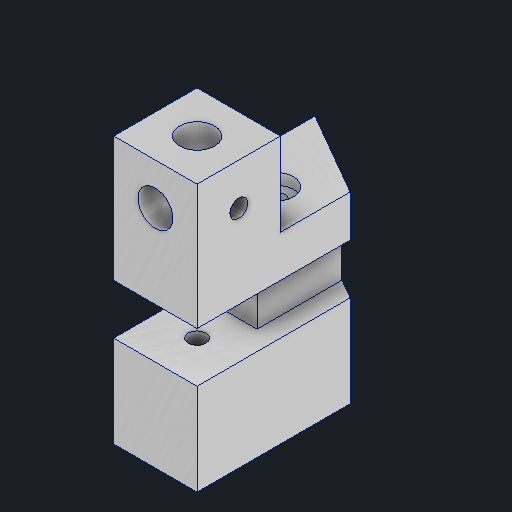
# Autodesk Inventor part: B Idler
Saved by Autodesk Inventor 2025.1 (Build 291241020, 241B)
## iProperties
Created: 2025-04-15
Part Number: B Idler
Material: Aluminum 6061
Document SubType Name: Modeling
Designer: Joshua Eah
Density: 2.7 g/cm^3
Appearance: Aluminum - Flat
Author: Joshua Eah
Autodesk Inventor part; units mm, degrees
ref_plane "YZ Plane" through (0, 0, 0) normal (1, 0, 0) x (0, 1, 0)
ref_plane "XZ Plane" through (0, 0, 0) normal (0, 1, 0) x (-1, 0, 0)
ref_plane "XY Plane" through (0, 0, 0) normal (0, 0, 1) x (1, 0, 0)
sketch "Sketch1" plane through (0, 0, 0) normal (0, 1, 0) x (-1, 0, 0)
  line L0 (0, 0) -> (-15, 0)
  line L1 (-15, 0) -> (-15, -36.2103)
  line L2 (-15, -36.2103) -> (0, -36.2103)
  line L3 (0, -36.2103) -> (0, 0)
  dimension "d0" = 15
  dimension "d1" = 36.2103
  constraints: 8 end point, 2 parallel, 1 horizontal, 1 perpendicular
  measures "d0" distance of L2.end L1.end
  measures "d1" distance of L1.end L0.end
extrude "Extrusion1" add sketch "Sketch1" along normal blind 48
sketch "Sketch2" plane through (0, 0, 0) normal (0, 0, 1) x (1, 0, 0)
  line L0 (0, 0) -> (15, 0) projected
  line L1 (15, 0) -> (15, 48) projected
  line L2 (0, 48) -> (15, 48) projected
  line L3 (0, 0) -> (0, 48) projected
  line L4 (0, 16.5) -> (3.5, 16.5)
  line L5 (3.5, 16.5) -> (3.5, 25.5)
  line L6 (3.5, 25.5) -> (0, 25.5)
  line L7 (0, 25.5) -> (0, 16.5)
  line L8 (15, 25.5) -> (11.5, 25.5)
  line L9 (11.5, 25.5) -> (11.5, 16.5)
  line L10 (11.5, 16.5) -> (15, 16.5)
  line L11 (15, 16.5) -> (15, 25.5)
  circle A0 centre (7.5, 40.5) radius 1.6
  line L12 (3.5, 16.5) -> (11.5, 16.5)
  line L13 (11.5, 16.5) -> (11.5, 25.5)
  line L14 (11.5, 25.5) -> (3.5, 25.5)
  line L15 (3.5, 25.5) -> (3.5, 16.5)
  point P0 (0, 25.5)
  dimension "d4" = 3.5
  dimension "d5" = 3.5
  dimension "d6" = 16.5
  dimension "d7" = 16.5
  dimension "d8" = 9
  dimension "d9" = 9
  dimension "d10" = 3.2
  dimension "d11" = 7.5
  dimension "d12" = 7.5
  constraints: 24 end point, 6 parallel, 3 horizontal, 3 perpendicular, 2 point on line, 1 centre point
  measures "d4" distance of L4.start L4.end
  measures "d5" distance of L9.end L10.end
  measures "d6" distance between parallel lines of L0 L4
  measures "d7" distance between parallel lines of L0 L10
  measures "d8" distance between parallel lines of L4 L6
  measures "d9" distance between parallel lines of L10 L8
  measures "d10" diameter of A0
  measures "d11" distance from line of L2 A0.centre
  measures "d12" distance from line of A0.centre L3
sketch "Sketch3" plane through (0, 48, 0) normal (0, 1, 0) x (1, 0, 0)
  line L0 (15, 0) -> (15, 36.2103) projected
  line L1 (0, 0) -> (15, 0)
  line L2 (15, 0) -> (15, 15)
  line L3 (15, 15) -> (0, 15)
  line L4 (0, 15) -> (0, 0)
  circle A0 centre (7.5, 7.5) radius 1.6
  line L5 (15, 36.2103) -> (0, 36.2103)
  line L6 (0, 36.2103) -> (0, 15)
  line L7 (0, 15) -> (15, 15)
  line L8 (15, 15) -> (15, 36.2103)
  dimension "d13" = 15
  dimension "d14" = 3.2
  dimension "d15" = 7.5
  dimension "d16" = 7.5
  constraints: 16 end point, 4 parallel, 2 horizontal, 2 perpendicular, 1 centre point, 1 point on line
  measures "d13" distance between parallel lines of L1 L3
  measures "d14" diameter of A0
  measures "d15" distance from line of A0.centre L4
  measures "d16" distance from line of A0.centre L1
extrude "Extrusion2" cut sketch "Sketch2" against normal through all contours L3 L6 L5 L4 | L10 L9 L8 L1
extrude "Extrusion3" cut sketch "Sketch2" against normal blind 14.3 contours L5 L14 L9 L12
extrude "Extrusion4" cut sketch "Sketch3" against normal blind 15 contours L3 L6 L5 L0
hole "Hole1" at (7.5, 40.5, 0) direction (0, 0, -1) diameter 3.2004 end through all counterbore diameter 6.2992 counterbore depth 12 clearance for "Oval Head Machine Screw" size "M3" standard "Ansi Metric M Profile"
hole "Hole2" at (7.5, 48, -7.5) direction (0, -1, 0) diameter 3.2004 end through all counterbore diameter 6.2992 counterbore depth 17 clearance for "Oval Head Machine Screw" size "M3" standard "Ansi Metric M Profile"
sketch "Sketch4" plane through (0, 25.5, 0) normal (-1, 0, 0) x (0, 0, 1)
  line L0 (-15, 22.5) -> (-15, 7.5) projected
  line L1 (-15, 7.5) -> (-36.2103, 7.5) projected
  line L2 (-36.2103, 0) -> (-36.2103, 7.5) projected
  line L3 (0, 0) -> (0, 22.5) projected
  line L4 (-15, 22.5) -> (0, 22.5) projected
  circle A0 centre (-7.5, 15) radius 1.6
  line L5 (-36.2103, -25.5) -> (0, -25.5) projected
  line L6 (0, -9) -> (-36.2103, -9) projected
  line L7 (-36.2103, -25.5) -> (-36.2103, -9) projected
  line L8 (0, -25.5) -> (0, -9) projected
  line L9 (-36.2103, 0) -> (0, 0) projected
  dimension "d37" = 3.2
  dimension "d38" = 7.5
  dimension "d39" = 7.5
  constraints: 1 centre point
  measures "d37" diameter of A0
  measures "d38" distance from line of A0.centre L0
  measures "d39" distance from line of L4 A0.centre
hole "Hole3" at (0, 40.5, -7.5) direction (1, 0, 0) diameter 3.2004 end through all counterbore diameter 6.2992 counterbore depth 12 clearance for "Oval Head Machine Screw" size "M3" standard "Ansi Metric M Profile"
sketch "Sketch5" plane through (0, 33, 0) normal (0, 1, 0) x (1, 0, 0)
  line L0 (15, 15) -> (0, 15) projected
  line L1 (15, 36.2103) -> (15, 15) projected
  line L2 (0, 36.2103) -> (15, 36.2103) projected
  line L3 (0, 15) -> (0, 36.2103) projected
  circle A0 centre (7.5, 21.7) radius 2.0546
  point P0 (0, 0)
  dimension "d47" = 7.5
  dimension "d48" = 6.7
  constraints: 1 centre point
  measures "d47" distance from line of A0.centre L3
  measures "d48" distance from line of A0.centre L0
hole "Hole4" at (7.5, 33, -21.7) direction (0, -1, 0) diameter 3.2004 end through all counterbore diameter 6.2992 counterbore depth 2 clearance for "Oval Head Machine Screw" size "M3" standard "Ansi Metric M Profile"
chamfer "Chamfer1" distance 15 angle 30 2 edges at (15, 8.25, -36.2103) (15, 29.25, -36.2103) measured on face at (14.5, 29.25, -36.2102) measured on face at (14.5, 8.25, -36.2102)
body "Solid1"
